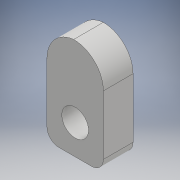
# Autodesk Inventor part: Clamp
Saved by Autodesk Inventor 2017 (Build 210142000, 142)
## iProperties
Created: 2016-12-07
Part Number: Clamp
Material: Generic
Document SubType Name: Modeling
Designer: willt
Density: 1 g/cm^3
Appearance: Default
Author: willt
Autodesk Inventor part; units mm, degrees
ref_plane "YZ Plane" through (0, 0, 0) normal (1, 0, 0) x (0, 1, 0)
ref_plane "XZ Plane" through (0, 0, 0) normal (0, 1, 0) x (-1, 0, 0)
ref_plane "XY Plane" through (0, 0, 0) normal (0, 0, 1) x (1, 0, 0)
sketch "Sketch1" plane through (0, 0, 0) normal (0, 1, 0) x (-1, 0, 0)
  line L0 (-4.75, 8.5) -> (4.75, 8.5)
  line L1 (4.75, 8.5) -> (4.75, -8.5)
  line L2 (4.75, -8.5) -> (-4.75, -8.5)
  line L3 (-4.75, -8.5) -> (-4.75, 8.5)
  line L4 (-4.75, 8.5) -> (4.75, -8.5) construction
  line L5 (4.75, 8.5) -> (-4.75, -8.5) construction
  line L6 (0, -8.5) -> (0, -3.5) construction
  circle A0 centre (0, -3.5) radius 2.25
  point P0 (0, 0)
  dimension "d2" = 9.5
  dimension "d3" = 17
  dimension "d4" = 5
  dimension "d5" = 4.5
  constraints: 14 end point, 3 midpoint, 2 parallel, 1 centre point, 1 coincident, 1 horizontal, 1 perpendicular, 1 vertical
  measures "d2" distance of L1.end L2.end
  measures "d3" distance of L0.end L1.end
  measures "d4" distance of L6.start L6.end
  measures "d5" diameter of A0
extrude "Extrusion1" add sketch "Sketch1" along normal blind 5
fillet "Fillet1" radius 5 1 edges at (4.75, 2.5, 8.5)
fillet "Fillet2" radius 5 1 edges at (-4.75, 2.5, 8.5)
fillet "Fillet3" radius 2 2 edges at (-4.75, 2.5, -8.5) (4.75, 2.5, -8.5)
body "Solid1"
